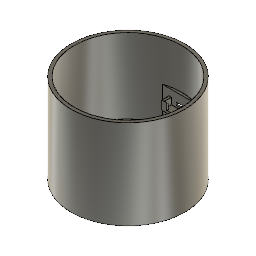
build-button-enclosure (Autodesk Fusion 360 design; units mm, degrees)
Autodesk Fusion 360 part; units mm, degrees
sketch "button-enclosure" plane through (0, 0, 0) normal (0, 0, 1) x (1, 0, 0)
  circle A0 centre (0, 0) radius 35
  circle A1 centre (0, 0) radius 33
  line L0 (-28.6278, 20.1357) -> (28.6278, 20.1357)
  line L1 (33.2711, -10.8643) -> (-33.2711, -10.8643)
  line L2 (-15.4609, 31.4) -> (15.4609, 31.4)
  line L3 (0, 0) -> (0, 35) construction
  dimension "d24" = 70
  dimension "d25" = 66
  dimension "d32" = 31
  dimension "d36" = 3.6
  measures "d24" diameter of A0
  measures "d25" diameter of A1
  measures "d32" distance of L0 L1
  measures "d36" distance of L2 A0.centre
extrude "Extrude9" add sketch "button-enclosure" along normal blind 55 contours A0 A1 L0 L1 | A0 A1 L0 L2 | A0 A1 L1 | A0 A1 L2 | A0 A1 L0 L1 | A0 A1 L0 L2
extrude "Extrude8" add sketch "button-enclosure" along normal blind 3
extrude "Extrude10" add sketch "button-enclosure" along normal blind 9 contours A1 L0 L2 | A1 L1 | A1 L2
extrude "Extrude11" add sketch "button-enclosure" along normal blind 30 contours A1 L2
ref_plane "WorkPlane3" through (0, 31.4, 19.5) normal (0, -1, 0) x (1, 0, 0)
ref_plane "WorkPlane4" through (0, 32.4, 19.5) normal (0, -1, 0) x (1, 0, 0)
sketch "flat-surface" plane through (0, 32.4, 32) normal (0, -1, 0) x (1, 0, 0)
  line L0 (8.5, -23.8701) -> (-8.5, -23.8701)
  line L1 (-11.5, -20.8701) -> (-11.5, -5.8701)
  line L2 (-8.5, -2.8701) -> (8.5, -2.8701)
  line L3 (11.5, -5.8701) -> (11.5, -20.8701)
  arc A0 (11.5, -5.8701) -> (8.5, -2.8701) centre (8.5, -5.8701) ccw
  arc A1 (-8.5, -2.8701) -> (-11.5, -5.8701) centre (-8.5, -5.8701) ccw
  arc A2 (8.5, -23.8701) -> (11.5, -20.8701) centre (8.5, -20.8701) ccw
  arc A3 (-11.5, -20.8701) -> (-8.5, -23.8701) centre (-8.5, -20.8701) ccw
  line L4 (35, -32) -> (-35, -32)
  line L5 (0, -32) -> (0, 8.7435) construction
  line L6 (3.5688, -18.24) -> (-3.59, -18.24)
  line L7 (-4.59, -19.24) -> (-4.59, -19.2996)
  line L8 (-2.09, -21.7996) -> (2.0688, -21.7996)
  line L9 (4.5688, -19.2996) -> (4.5688, -19.24)
  arc A4 (2.0688, -21.7996) -> (4.5688, -19.2996) centre (2.0688, -19.2996) ccw
  arc A5 (-4.59, -19.2996) -> (-2.09, -21.7996) centre (-2.09, -19.2996) ccw
  arc A6 (4.5688, -19.24) -> (3.5688, -18.24) centre (3.5688, -19.24) ccw
  arc A7 (-3.59, -18.24) -> (-4.59, -19.24) centre (-3.59, -19.24) ccw
  line L10 (-1.85, -9.0168) -> (1.85, -9.0168)
  line L11 (1.85, -9.0168) -> (1.85, -7.3168)
  line L12 (1.85, -7.3168) -> (-1.85, -7.3168)
  line L13 (-1.85, -7.3168) -> (-1.85, -9.0168)
  line L14 (-1.85, -9.0168) -> (1.85, -7.3168) construction
  line L15 (1.85, -9.0168) -> (-1.85, -7.3168) construction
  line L16 (4.675, -6.1668) -> (-4.675, -6.1668)
  line L17 (-4.675, -6.1668) -> (-4.675, -10.1668)
  line L18 (-4.675, -10.1668) -> (4.675, -10.1668)
  line L19 (4.675, -10.1668) -> (4.675, -6.1668)
  line L20 (4.675, -6.1668) -> (-4.675, -10.1668) construction
  line L21 (-4.675, -6.1668) -> (4.675, -10.1668) construction
  line L22 (-4.675, -6.1668) -> (-6.175, -6.1668)
  line L23 (-6.175, -6.1668) -> (-6.175, -11.6668)
  line L24 (-6.175, -11.6668) -> (6.175, -11.6668)
  line L25 (6.175, -11.6668) -> (6.175, -6.1668)
  line L26 (6.175, -6.1668) -> (4.675, -6.1668)
  line L27 (-3.175, -6.1668) -> (-3.175, -10.1668)
  line L28 (3.175, -6.1668) -> (3.175, -10.1668)
  point P0 (-20, 0)
  dimension "d43" = 3
  dimension "d44" = 3
  dimension "d45" = 3
  dimension "d46" = 3
  dimension "d49" = 21
  dimension "d50" = 23
  dimension "d51" = 2.5
  dimension "d54" = 1
  dimension "d55" = 1
  dimension "d78" = 3.7
  dimension "d79" = 1.7
  dimension "d82" = 9.35
  dimension "d83" = 4
  dimension "d84" = 1.5
  dimension "d85" = 1.5
  dimension "d86" = 1.5
  dimension "d87" = 1.5
  dimension "d88" = 1.5
  measures "d43" radius of A0
  measures "d44" radius of A1
  measures "d45" radius of A2
  measures "d46" radius of A3
  measures "d49" distance of L0 L2
  measures "d50" distance of L1 L3
  measures "d51" radius of A4
  measures "d54" radius of A6
  measures "d55" radius of A7
  measures "d84" distance of L17 L23
  measures "d85" distance of L18 L24
  measures "d86" distance of L19 L25
  measures "d87" distance of L17 L27
  measures "d88" distance of L19 L28
ref_plane "WorkPlane6" through (0, 28, 32) normal (0, -1, 0) x (1, 0, 0)
extrude "Extrude19" cut sketch "flat-surface" along normal blind 4 contours L10 L11 L12 L13
extrude "Extrude12" cut sketch "flat-surface" against normal blind 17 contours L0 L1 L2 L3 A0 A1 A2 A3 | L6 L7 L8 L9 A4 A5 A6 A7 | L10 L11 L12 L13 | L16 L18 L19 L28 | L17 L18 L19 L22 L23 L24 L25 L26 | L16 L18 L27 L28 | L16 L17 L18 L27
extrude "Extrude13" cut sketch "flat-surface" along normal blind 4 contours L6 L7 L8 L9 A4 A5 A6 A7
ref_plane "WorkPlane5" through (0, 0, 105) normal (0, 0, 1) x (1, 0, 0)
sketch "feather-mounting-holes" plane through (0, 0, 9) normal (0, 0, 1) x (-1, 0, 0)
  line L0 (-10.1509, -31.4) -> (10.1509, -31.4)
  arc A0 (10.1509, -31.4) -> (26.1449, -20.1357) centre (0, 0) ccw
  line L1 (26.1449, -20.1357) -> (-26.1449, -20.1357)
  arc A1 (-26.1449, -20.1357) -> (-10.1509, -31.4) centre (0, 0) ccw
  circle A2 centre (8.89, -28.6978) radius 1.3
  circle A3 centre (-8.89, -28.653) radius 1.3
  circle A4 centre (8.89, 17.1572) radius 1.3
  circle A5 centre (-8.89, 17.0677) radius 1.3
  dimension "d72" = 2.6
  dimension "d73" = 2.6
  dimension "d74" = 2.6
  dimension "d75" = 2.6
  measures "d72" diameter of A2
  measures "d73" diameter of A3
  measures "d74" diameter of A4
  measures "d75" diameter of A5
extrude "Extrude18" cut sketch "feather-mounting-holes" against normal blind 8 contours A2 | A3 | A4 | A5
extrude "Extrude20" add sketch "flat-surface" along normal blind 4.4 contours L17 L18 L19 L22 L23 L24 L25 L26
sketch "switch-holder-lip" plane through (0, 28, 32) normal (0, -1, 0) x (1, 0, 0)
  line L0 (-3.175, -6.1668) -> (-3.175, -10.1668)
  line L1 (-6.175, -6.1668) -> (-3.175, -6.1668)
  line L2 (-3.175, -10.1668) -> (3.175, -10.1668)
  line L3 (4.675, -6.1668) -> (-4.675, -6.1668)
  line L4 (3.175, -10.1668) -> (3.175, -6.1668)
  line L5 (-6.175, -11.6668) -> (6.175, -11.6668)
  line L6 (6.175, -6.1668) -> (6.175, -11.6668)
  line L7 (-6.175, -11.6668) -> (-6.175, -6.1668)
  line L8 (4.675, -6.1668) -> (6.175, -6.1668)
extrude "Extrude21" add sketch "switch-holder-lip" along normal blind 1 contours L0 L1 L2 L3 L4 L5 L6 L7 L8
fillet "Fillet3" radius 2 2 edges at (3.925, 28, 25.8332) (-3.925, 28, 25.8332)
chamfer "Chamfer1" distance 4.4 angle 45 1 edges at (0, 31.4, 20.3332)
named bodies: "enclosure"
